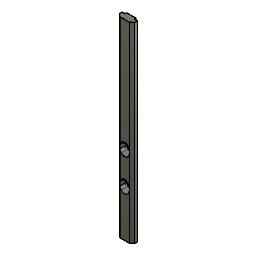
base-spacer (Autodesk Fusion 360 design; units mm, degrees)
Autodesk Fusion 360 part; units mm, degrees
sketch "BaseProfile" plane through (0, 0, 0) normal (0, 1, 0) x (1, 0, 0)
  line L0 (-2.875, 0) -> (2.875, 0)
  line L1 (2.875, 0) -> (2.875, -1)
  line L2 (2.875, -1) -> (4.75, -1)
  line L3 (2.875, -4.25) -> (-2.875, -4.25)
  line L4 (-4.75, -1) -> (-2.875, -1)
  line L5 (-2.875, -1) -> (-2.875, 0)
  line L6 (-4.75, -1) -> (-4.75, -2.75)
  line L7 (-4.75, -2.75) -> (-2.875, -4.25)
  line L8 (4.75, -1) -> (4.75, -2.75)
  line L9 (4.75, -2.75) -> (2.875, -4.25)
  line L10 (0, 7.3711) -> (0, -7.6289)
  dimension "d1" = 5.75
  dimension "d2" = 5.75
  dimension "d3" = 9.5
  dimension "d4" = 1
  dimension "d7" = 1.75
  dimension "d8" = 1.5
  constraint perpendicular L0 L1
  constraint perpendicular L1 L2
  constraint perpendicular L1 L3
  constraint parallel L3 L4
  constraint perpendicular L0 L5
  constraint perpendicular L4 L6
  constraint perpendicular L2 L8
  constraint vertical L10
  constraint symmetric L0.start L0.end L10
  constraint symmetric L2.end L4.start L10
  constraint vertical L0.start L3.end
  constraint collinear origin L10.start L10.end
  constraint horizontal L6.end L8.end
  constraint horizontal origin L0.start
  measures "d1" distance of L0.start L0.end
  measures "d2" distance of L3.start L3.end
  measures "d3" distance of L2.end L4.start
  measures "d4" distance of L0.start L4.end
  measures "d7" distance of L4.start L6.end
  measures "d8" vertical distance of L3.end L6.end
extrude "4mmExt" add sketch "BaseProfile" along normal blind 4 makes body 1
extrude "104mmExt" add sketch "BaseProfile" along normal blind 104 separate body makes body 2
extrude "139mmExt" add sketch "BaseProfile" along normal blind 139 separate body makes body 3
extrude "24mmExt" add sketch "BaseProfile" along normal blind 24 separate body makes body 4
extrude "94mmExt (1)" add sketch "BaseProfile" along normal blind 94 separate body makes body 5
sketch "14mm34mm" plane through (0, 0, 0) normal (0, 0, 1) x (1, 0, 0)
  line L0 (-2.875, 15) -> (-2.875, 13)
  arc A0 (-2.875, 13) -> (2.875, 13) centre (0, 13) ccw
  line L1 (2.875, 13) -> (2.875, 15)
  arc A1 (2.875, 15) -> (-2.875, 15) centre (0, 15) ccw
  line L2 (0, 15) -> (0, 13) construction
  line L3 (-2.875, 35) -> (-2.875, 33)
  arc A2 (-2.875, 33) -> (2.875, 33) centre (0, 33) ccw
  line L4 (2.875, 33) -> (2.875, 35)
  arc A3 (2.875, 35) -> (-2.875, 35) centre (0, 35) ccw
  line L5 (0, 35) -> (0, 33) construction
  point P0 (0, 14)
  point P1 (0, 34)
  dimension "d19" = 5.75
  dimension "d20" = 14
  dimension "d21" = 1
  dimension "d42" = 5.75
  dimension "d43" = 20
  dimension "d44" = 1
  constraint tangent L0 A0
  constraint tangent A0 L1
  constraint parallel L0 L1
  constraint tangent L1 A1
  constraint tangent L0 A1
  constraint vertical L2
  constraint midpoint L2 P0
  constraint vertical P0 origin
  constraint tangent L3 A2
  constraint tangent A2 L4
  constraint parallel L3 L4
  constraint tangent L4 A3
  constraint tangent L3 A3
  constraint vertical L5
  constraint midpoint L5 P1
  constraint vertical P0 P1
  measures "d19" diameter of A0
  measures "d20" distance of P0 origin
  measures "d21" distance of A0.centre P0
  measures "d42" diameter of A2
  measures "d43" distance of P0 P1
  measures "d44" distance of A2.centre P1
extrude "14mm34mmCut" cut sketch "14mm34mm" along normal through all bodies 5
extrude "Extrude7" add sketch "BaseProfile" along normal blind 119 separate body makes body 6
sketch "29mm49mm" plane through (0, 0, 0) normal (0, 0, 1) x (1, 0, 0)
  line L0 (-2.875, 30) -> (-2.875, 28)
  arc A0 (-2.875, 28) -> (2.875, 28) centre (0, 28) ccw
  line L1 (2.875, 28) -> (2.875, 30)
  arc A1 (2.875, 30) -> (-2.875, 30) centre (0, 30) ccw
  line L2 (0, 30) -> (0, 28) construction
  line L3 (-2.875, 50) -> (-2.875, 48)
  arc A2 (-2.875, 48) -> (2.875, 48) centre (0, 48) ccw
  line L4 (2.875, 48) -> (2.875, 50)
  arc A3 (2.875, 50) -> (-2.875, 50) centre (0, 50) ccw
  line L5 (0, 50) -> (0, 48) construction
  point P0 (0, 29)
  point P1 (0, 49)
  dimension "d27" = 5.75
  dimension "d28" = 1
  dimension "d29" = 29
  dimension "d30" = 5.75
  dimension "d31" = 20
  dimension "d32" = 1
  constraint tangent L0 A0
  constraint tangent A0 L1
  constraint parallel L0 L1
  constraint tangent L1 A1
  constraint tangent L0 A1
  constraint vertical L2
  constraint midpoint L2 P0
  constraint vertical P0 origin
  constraint tangent L3 A2
  constraint tangent A2 L4
  constraint parallel L3 L4
  constraint tangent L4 A3
  constraint tangent L3 A3
  constraint vertical L5
  constraint midpoint L5 P1
  constraint vertical P0 P1
  measures "d27" diameter of A0
  measures "d28" distance of A0.centre P0
  measures "d29" distance of P0 origin
  measures "d30" diameter of A2
  measures "d31" distance of P0 P1
  measures "d32" distance of A2.centre P1
extrude "29mm49mmCut" cut sketch "29mm49mm" along normal through all bodies 6
extrude "23mmExt" add sketch "BaseProfile" along normal blind 24 separate body makes body 7
sketch "14mm" plane through (0, 0, 0) normal (0, 0, 1) x (1, 0, 0)
  line L0 (-2.875, 15) -> (-2.875, 13)
  arc A0 (-2.875, 13) -> (2.875, 13) centre (0, 13) ccw
  line L1 (2.875, 13) -> (2.875, 15)
  arc A1 (2.875, 15) -> (-2.875, 15) centre (0, 15) ccw
  line L2 (0, 15) -> (0, 13) construction
  point P0 (0, 14)
  dimension "d36" = 5.75
  dimension "d37" = 1
  dimension "d38" = 14
  constraint tangent L0 A0
  constraint tangent A0 L1
  constraint parallel L0 L1
  constraint tangent L1 A1
  constraint tangent L0 A1
  constraint vertical L2
  constraint midpoint L2 P0
  constraint vertical P0 origin
  measures "d36" diameter of A0
  measures "d37" distance of A0.centre P0
  measures "d38" distance of P0 origin
extrude "14mmCut" cut sketch "14mm" along normal through all bodies 7
extrude "94mmExt" add sketch "BaseProfile" along normal blind 94 separate body makes body 8
hidden bodies 1 2 3 4 5 7 8
equation "d8 = 3.25 mm - 1.75 mm"
named bodies: "4mm", "104mm", "139mm", "24mm", "94mmSlot14mmSlot34", "119mmSlot29Slot49", "23mmSlot14mm", "94mm"
